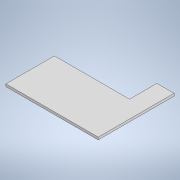
# Autodesk Inventor part: board_R
Saved by Autodesk Inventor 2020 (Build 240168000, 168)
## iProperties
Created: 2022-07-25
Part Number: board_R
Material: 일반
Document SubType Name: Modeling
Designer: SeungJin
Density: 1 g/cm^3
Appearance: 기본값
Author: SeungJin
Autodesk Inventor part; units mm, degrees
ref_plane "YZ Plane" through (0, 0, 0) normal (1, 0, 0) x (0, 1, 0)
ref_plane "XZ Plane" through (0, 0, 0) normal (0, 1, 0) x (-1, 0, 0)
ref_plane "XY Plane" through (0, 0, 0) normal (0, 0, 1) x (1, 0, 0)
ref_plane "작업 평면1" through (150.5, 0, 75) normal (0, 1, 0) x (1, 0, 0)
sketch "스케치1" plane through (150.5, 0, 75) normal (0, 1, 0) x (1, 0, 0)
  line L0 (75, -152.5) -> (-110.5, -152.5)
  line L1 (75, 0) -> (75, -152.5)
  line L2 (0, 0) -> (75, 0)
  line L3 (0, 10) -> (0, 0)
  line L4 (-110.5, 10) -> (0, 10)
  line L5 (-110.5, -152.5) -> (-110.5, 10)
  line L6 (-110.5, 10) -> (0, 10)
  line L7 (-110.5, 10) -> (40.5, 10)
  line L8 (40.5, 10) -> (40.5, -55)
  line L9 (40.5, -55) -> (-110.5, -55)
  line L10 (-110.5, -55) -> (-110.5, 10)
  point P0 (-150.5, 75)
  point P1 (40.5, 0)
  point P2 (-110.5, -55)
  dimension "d1" = 151
  dimension "d2" = 65
  constraints: 22 end point
  measures "d1" distance of L8.end L9.end
  measures "d2" distance of L7.end L8.end
extrude "돌출1" add sketch "스케치1" along normal blind 5 contours L0 L5 L9 L8 L2 L1
